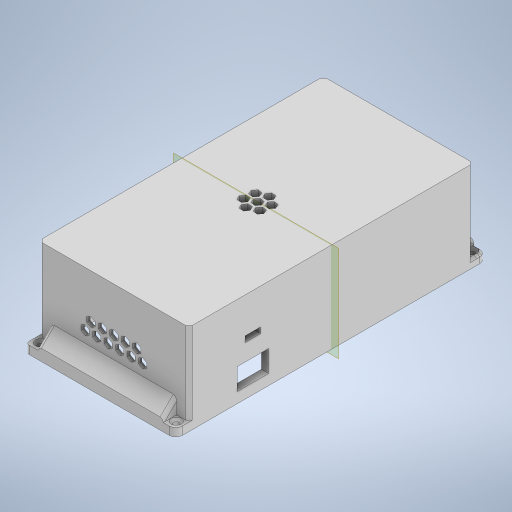
# Autodesk Inventor part: electronics-mount
Saved by Autodesk Inventor 2024.2 (Build 282272000, 272)
## iProperties
Created: 2024-02-05
Part Number: electronics-mount
Material: Generic
Document SubType Name: Modeling
Designer: crow
Density: 1 g/cm^3
Appearance: Default
Author: crow
## iProperties of the stored document electronics-mount_3DPrint.ipt
Created: 2024-02-08
Part Number: electronics-mount_3DPrint
Material: Generic
Document SubType Name: Modeling
Designer: crow
Density: 1 g/cm^3
Appearance: Default
Author: crow
Autodesk Inventor part; units mm, degrees
ref_plane "YZ Plane" through (0, 0, 0) normal (1, 0, 0) x (0, 1, 0)
ref_plane "XZ Plane" through (0, 0, 0) normal (0, 1, 0) x (-1, 0, 0)
ref_plane "XY Plane" through (0, 0, 0) normal (0, 0, 1) x (1, 0, 0)
sketch "Sketch1" plane through (0, 0, 0) normal (0, 1, 0) x (-1, 0, 0)
  line L0 (-41.6915, 94.55) -> (43.6915, 94.55)
  line L1 (45.6915, 92.55) -> (45.6915, -90.55)
  line L2 (41.6915, -94.55) -> (-41.6915, -94.55)
  line L3 (-45.6915, -90.55) -> (-45.6915, 90.55)
  line L4 (41.305, 89.8895) -> (-41.305, 89.8895) construction
  line L5 (0, 89.8895) -> (0, -90.716948) construction
  line L6 (62.379819, 0) -> (-60.787127, 0) construction
  line L7 (41.305, 89.8895) -> (41.305, -89.8895) construction
  line L8 (41.305, 0) -> (-44.332283, 0) construction
  arc A0 (45.6915, 92.55) -> (43.6915, 94.55) centre (43.6915, 92.55) ccw
  arc A1 (41.6915, -94.55) -> (45.6915, -90.55) centre (41.6915, -90.55) ccw
  arc A2 (-45.6915, -90.55) -> (-41.6915, -94.55) centre (-41.6915, -90.55) ccw
  arc A3 (-41.6915, 94.55) -> (-45.6915, 90.55) centre (-41.6915, 90.55) ccw
  line L9 (41.3045, 84.55) -> (-41.3045, 84.55)
  line L10 (-41.3045, 84.55) -> (-41.3045, -84.55)
  line L11 (-41.3045, -84.55) -> (41.3045, -84.55)
  line L12 (41.3045, -84.55) -> (41.3045, 84.55)
  point P0 (0, 0)
  point P1 (45.6915, -94.55)
  point P2 (45.6915, 94.55)
  point P3 (-45.6915, -94.55)
  point P4 (-41.305, -89.8895)
  dimension "d0" = 91.383
  dimension "d1" = 189.1
  dimension "d2" = 82.61
  dimension "d3" = 179.779
  dimension "d4" = 82.61
  dimension "d5" = 2
  dimension "d6" = 4
  dimension "d16" = 10
  dimension "d17" = 4.387
  dimension "d18" = 10
  dimension "d19" = 4.387
  constraints: 26 end point, 8 point on circle, 8 point on line, 8 tangent, 5 horizontal, 4 centre point, 4 parallel, 2 coincident, 2 equal radius, 2 midpoint, 2 perpendicular, 2 vertical
  measures "d0" distance of point (45.691, -94.55) point (-45.691, -94.55)
  measures "d1" distance of point (45.691, 94.55) point (45.691, -94.55)
  measures "d2" distance of L4.start L4.end
  measures "d3" distance of L4.start L7.end
  measures "d4" distance of point (41.305, -89.889) point (-41.305, -89.889)
  measures "d5" radius of A0
  measures "d6" radius of A1
  measures "d16" distance between parallel lines of L0 L9
  measures "d17" distance between parallel lines of L1 L12
  measures "d18" distance between parallel lines of L2 L11
  measures "d19" distance between parallel lines of L3 L10
extrude "Extrusion1" add sketch "Sketch1" against normal blind 5
hole "Hole1" at (-41.305, 0, 89.8895) at (41.305, 0, 89.8895) at (-41.305, 0, -89.8895) at (41.305, 0, -89.8895) direction (0, -1, 0) diameter 3.4 depth 5 countersink diameter 6.3 countersink angle 90 clearance for "Countersunk Flat Head Screw ISO 2009/7046" size "M3" standard "ISO"
sketch "Sketch2" plane through (0, 0, 0) normal (0, 1, 0) x (1, 0, 0)
  line L0 (-41.3045, -84.55) -> (-41.3045, 84.55)
  line L1 (41.3045, -84.55) -> (-41.3045, -84.55)
  line L2 (41.3045, 84.55) -> (41.3045, -84.55)
  line L3 (-41.3045, 84.55) -> (41.3045, 84.55)
  line L4 (-43.6915, -86.55) -> (43.6915, -86.55)
  line L5 (45.6915, -84.55) -> (45.6915, 84.710496)
  line L6 (43.6915, 86.710496) -> (-43.6915, 86.710496)
  line L7 (-45.6915, 84.710496) -> (-45.6915, -84.55)
  line L8 (-43.6915, -86.55) -> (-45.6915, -84.55)
  line L9 (-45.6915, 84.710496) -> (-43.6915, 86.710496)
  line L10 (45.6915, 84.710496) -> (43.6915, 86.710496)
  line L11 (45.6915, -84.55) -> (43.6915, -86.55)
  line L12 (45.6915, -90.55) -> (45.6915, 90.55)
  line L13 (-45.6915, 90.55) -> (-45.6915, -92.55)
  point P0 (0, 0)
  point P1 (-45.6915, -86.55)
  point P2 (-45.6915, 86.710496)
  point P3 (45.6915, 86.710496)
  point P4 (45.6915, -86.55)
  dimension "d20" = 2
  dimension "d24" = 2
  dimension "d25" = 2
  dimension "d26" = 2
  dimension "d27" = 2
  dimension "d28" = 2
  dimension "d29" = 2
  dimension "d30" = 2
  dimension "d31" = 2
  constraints: 16 end point, 8 point on line, 2 collinear
  measures "d20" distance between parallel lines of L1 L4
  measures "d24" distance of L4.start point (-45.692, -86.55)
  measures "d25" distance of L7.end point (-45.692, -86.55)
  measures "d26" distance of L7.start point (-45.692, 86.71)
  measures "d27" distance of L6.end point (-45.692, 86.71)
  measures "d28" distance of L5.end point (45.691, 86.71)
  measures "d29" distance of L6.start point (45.691, 86.71)
  measures "d30" distance of L5.start point (45.691, -86.55)
  measures "d31" distance of L4.end point (45.691, -86.55)
extrude "Extrusion2" add sketch "Sketch2" along normal blind 40
sketch "Sketch3" plane through (0, 40, 0) normal (0, 1, 0) x (1, 0, 0)
  line L0 (-45.6915, -84.55) -> (-43.6915, -86.55)
  line L1 (-43.6915, -86.55) -> (43.6915, -86.55)
  line L2 (43.6915, -86.55) -> (45.6915, -84.55)
  line L3 (45.6915, -84.55) -> (45.6915, 84.710496)
  line L4 (45.6915, 84.710496) -> (43.6915, 86.710496)
  line L5 (43.6915, 86.710496) -> (-43.6915, 86.710496)
  line L6 (-43.6915, 86.710496) -> (-45.6915, 84.710496)
  line L7 (-45.6915, 84.710496) -> (-45.6915, -84.55)
  line L8 (-41.3045, -84.55) -> (-41.3045, 84.55)
  line L9 (-41.3045, 84.55) -> (41.3045, 84.55)
  line L10 (41.3045, 84.55) -> (41.3045, -84.55)
  line L11 (41.3045, -84.55) -> (-41.3045, -84.55)
  point P0 (0, 0)
extrude "Extrusion3" add sketch "Sketch3" along normal blind 10 contours L7 L6 L5 L4 L3 L2 L1 L0 | L8 L9 L10 L11
sketch "Sketch4" plane through (0, 40, 0) normal (0, -1, 0) x (1, 0, 0)
  line L0 (-41.3045, -84.55) -> (-41.3045, 84.55)
  line L1 (-41.3045, 84.55) -> (41.3045, 84.55)
  line L2 (41.3045, -84.55) -> (-41.3045, -84.55)
  line L3 (40.8045, 67.80558) -> (-34.1955, 67.80558)
  line L4 (-34.1955, 67.80558) -> (-34.1955, 29.80558)
  line L5 (-34.1955, 29.80558) -> (40.8045, 29.80558)
  line L6 (40.8045, 29.80558) -> (40.8045, 67.80558)
  line L7 (41.3045, 84.55) -> (41.3045, -84.55)
  circle A0 centre (-29.1955, 62.80558) radius 2
  line L8 (-34.1955, 48.80558) -> (40.8045, 48.80558)
  line L9 (3.3045, 67.80558) -> (3.3045, 29.80558)
  circle A1 centre (-29.1955, 34.80558) radius 2
  line L10 (3.3045, 29.80558) -> (3.3045, 67.80558)
  circle A2 centre (35.8045, 62.80558) radius 2
  circle A3 centre (35.8045, 34.80558) radius 2
  line L11 (29, -27.05) -> (-29, -27.05)
  line L12 (-29, -27.05) -> (-29, -82.55)
  line L13 (-29, -82.55) -> (29, -82.55)
  line L14 (29, -82.55) -> (29, -27.05)
  line L15 (0, -27.05) -> (0, -82.55) construction
  line L16 (-29, -54.8) -> (29, -54.8) construction
  line L17 (0, 99.928537) -> (0, -124.554691) construction
  circle A4 centre (24.5, -37.55) radius 2
  circle A5 centre (24.5, -72.05) radius 2
  circle A6 centre (-15.5, -48.55) radius 2
  circle A7 centre (-15.5, -61.05) radius 2
  line L18 (35, 18.5) -> (-35, 18.5)
  line L19 (-35, 18.5) -> (-35, -18.5)
  line L20 (-35, -18.5) -> (35, -18.5)
  line L21 (35, -18.5) -> (35, 18.5)
  line L22 (0, 18.5) -> (0, -18.5) construction
  line L23 (35, 0) -> (-35, 0) construction
  line L24 (74.043024, 0) -> (-69.253155, 0) construction
  circle A8 centre (0, -25) radius 2
  line L25 (0, -25) -> (0, 25)
  circle A9 centre (0, 25) radius 2
  line L26 (0, 0) -> (13.891236, 0)
  dimension "d123" = 75
  dimension "d124" = 38
  dimension "d125" = 0.5
  dimension "d126" = 4
  dimension "d129" = 58
  dimension "d130" = 55.5
  dimension "d131" = 2
  dimension "d132" = 4
  dimension "d133" = 5
  dimension "d134" = 5
  dimension "d135" = 10.5
  dimension "d136" = 4.5
  dimension "d138" = 4.5
  dimension "d139" = 34.5
  dimension "d140" = 13.5
  dimension "d141" = 21.5
  dimension "d142" = 13.5
  dimension "d143" = 12.5
  dimension "d144" = 70
  dimension "d145" = 37
  dimension "d153" = 4
  dimension "d154" = 50
  dimension "d155" = 4
  constraints: 46 end point, 13 midpoint, 10 centre point, 6 horizontal, 6 parallel, 5 symmetric about line, 4 collinear, 3 equal radius, 3 perpendicular, 2 point on line, 2 vertical, 1 coincident, 3 other
  measures "d123" distance of L5.end L4.end
  measures "d124" distance of L4.end L3.end
  measures "d125" distance between parallel lines of L7 L6
  measures "d126" diameter of A0
  measures "d129" distance of L13.end L12.end
  measures "d130" distance of L12.end L11.end
  measures "d131" distance between parallel lines of L2 L13
  measures "d132" diameter of A4
  measures "d133" distance from line of L3 A0.centre
  measures "d134" distance from line of L4 A0.centre
  measures "d135" distance from line of L11 A4.centre
  measures "d136" distance from line of L14 A4.centre
  measures "d138" distance from line of L14 A5.centre
  measures "d139" distance of A4.centre A5.centre
  measures "d140" distance from line of L12 A6.centre
  measures "d141" distance from line of L11 A6.centre
  measures "d142" distance from line of L12 A7.centre
  measures "d143" distance of A7.centre A6.centre
  measures "d144" distance of L20.end L19.end
  measures "d145" distance of L19.end L18.end
  measures "d153" diameter of A8
  measures "d154" distance of L25.start L25.end
  measures "d155" diameter of A9
extrude "Extrusion4" cut sketch "Sketch4" against normal blind 8.2 contours A0 | A1 | A2 | A3 | A4 | A5 | A6 | A7 | A8 | A9
sketch "Sketch5" plane through (0, 0, 0) normal (0, 1, 0) x (1, 0, 0)
  line L0 (-41.6915, 94.55) -> (41.6915, 94.55) projected
  line L1 (38.155, 94.55) -> (-38.155, 94.55)
  line L2 (-38.155, 94.55) -> (-38.155, 86.7395)
  line L3 (-38.155, 86.7395) -> (38.155, 86.7395)
  line L4 (38.155, 86.7395) -> (38.155, 94.55)
  circle A0 centre (41.305, 89.8895) radius 3.15 projected
  point P0 (0, 0)
  constraints: 8 end point, 2 parallel, 1 horizontal, 1 perpendicular, 1 point on line, 1 tangent
extrude "Extrusion5" add sketch "Sketch5" along normal blind 10 contours L0 L4 L3 L2
chamfer "Chamfer4" distance 7.81 angle 45 1 edges at (0, 10, -94.55)
chamfer "Chamfer5" distance 1.5 angle 45 6 edges at (-45.6915, 0, -87.6302) (-44.5199, 0, -93.3784) (-39.9232, 0, -94.55) (44.5199, 0, -93.3784) (39.9233, 0, -94.55) (45.6915, 0, -87.6302)
fillet "Fillet1" radius 2 2 edges at (38.155, 6.095, -90.645) (-38.155, 6.095, -90.645)
ref_plane "Work Plane2" through (43.6915, 0, -0.080248) normal (0, 0, -1) x (-1, 0, 0)
mirror "Mirror1" about plane through (43.6915, 0, -0.080248) normal (0, 0, -1) of "Extrusion5", "Fillet1", "Chamfer4"
move faces "Move1" translate (0, 0, 0.160496) faces at (12.051667, 0.73, 94.389504)
sketch "Sketch7" plane through (45.6915, -5, 90.55) normal (1, 0, 0) x (0, 0, -1)
  line L0 (175.1, 45) -> (6, 45)
  line L1 (181.1, 0) -> (0, 0)
  line L2 (6, 5) -> (6, 55)
  line L3 (57.74442, 45) -> (53.74442, 45)
  line L4 (29.74442, 45) -> (25.74442, 45)
  line L5 (29.74442, 53.2) -> (25.74442, 53.2)
  line L6 (57.74442, 53.2) -> (53.74442, 53.2)
  line L7 (55.74442, 53.2) -> (55.74442, 64.703518)
  line L8 (27.74442, 53.2) -> (27.74442, 64.703518)
  line L9 (55.74442, 45) -> (55.74442, 35)
  line L10 (55.74442, 35) -> (27.74442, 35)
  line L11 (27.74442, 35) -> (27.74442, 45)
  line L12 (55.74442, 35) -> (55.74442, 33.4)
  line L13 (55.74442, 33.4) -> (27.74442, 33.4)
  line L14 (27.74442, 33.4) -> (27.74442, 35)
  line L15 (47.54442, 29.9) -> (38.24442, 29.9)
  line L16 (38.24442, 29.9) -> (38.24442, 33.4)
  line L17 (38.24442, 33.4) -> (47.54442, 33.4)
  line L18 (47.54442, 33.4) -> (47.54442, 29.9)
  line L19 (52.49442, 19.6) -> (33.29442, 19.6)
  line L20 (33.29442, 19.6) -> (33.29442, 6.4)
  line L21 (33.29442, 6.4) -> (52.49442, 6.4)
  line L22 (52.49442, 6.4) -> (52.49442, 19.6)
  line L23 (42.89442, 6.4) -> (42.89442, 19.6) construction
  line L24 (52.49442, 13) -> (33.29442, 13) construction
  point P0 (90.55, 5)
  point P1 (38.24442, 31.65)
  point P2 (47.54442, 31.65)
  point P3 (47.54442, 33.4)
  point P4 (40, 13)
  point P5 (42.89442, 13)
  point P6 (42.89442, 29.9)
  dimension "d156" = 10
  dimension "d157" = 28
  dimension "d158" = 1.6
  dimension "d160" = 8.2
  dimension "d161" = 9.3
  dimension "d162" = 3.5
  dimension "d166" = 19.2
  dimension "d167" = 13.2
  dimension "d170" = 16.9
  dimension "d171" = 0
  constraints: 36 end point, 12 midpoint, 4 parallel, 4 perpendicular, 4 vertical, 2 collinear, 2 horizontal
  measures "d156" distance of L9.start L9.end
  measures "d157" distance of L9.end L10.end
  measures "d158" distance of L9.end L12.end
  measures "d160" distance from line of L9 point (47.544, 31.65)
  measures "d161" distance of L15.start L15.end
  measures "d162" distance of L15.end L16.end
  measures "d166" distance of L21.end L20.end
  measures "d167" distance of L20.end L19.end
  measures "d170" distance from line of L15 point (42.894, 13)
  measures "d171" distance from line of point (42.894, 29.9) L23
extrude "Extrusion7" cut sketch "Sketch7" against normal blind 10 contours L18 L15 L16 L13 | L22 L21 L20 L19
sketch "Sketch6" plane through (-45.6915, -5, 92.55) normal (-1, 0, 0) x (0, 0, 1)
  circle A0 centre (-44.89442, 13) radius 6.2
  line L0 (-8, 45) -> (-177.1, 45)
  line L1 (-8, 5) -> (-8, 55)
  line L2 (-54.49442, 6.4) -> (-54.49442, 19.6)
  line L3 (-35.29442, 19.6) -> (-35.29442, 6.4)
  line L4 (-35.29442, 6.4) -> (-54.49442, 6.4)
  line L5 (-54.49442, 19.6) -> (-35.29442, 19.6)
  line L6 (-44.89442, 6.4) -> (-44.89442, 19.6) construction
  line L7 (-54.49442, 13) -> (-35.29442, 13) construction
  point P0 (-92.55, 5)
  dimension "d96" = 12.4
  dimension "d97" = 32
  constraints: 5 midpoint, 4 end point, 1 centre point
  measures "d96" diameter of A0
  measures "d97" distance from line of L0 A0.centre
extrude "Extrusion6" cut sketch "Sketch6" against normal blind 10 contours A0
sketch "Sketch8" plane through (0, 50, 0) normal (0, 1, 0) x (1, 0, 0)
  circle A0 centre (-16.5, -72.55) radius 2
  circle A1 centre (16.5, -72.55) radius 2
  line L0 (-43.6915, -86.55) -> (43.6915, -86.55)
  line L1 (43.6915, -86.55) -> (45.6915, -84.55)
  line L2 (45.6915, -84.55) -> (45.6915, 84.710496)
  line L3 (45.6915, 84.710496) -> (43.6915, 86.710496)
  line L4 (43.6915, 86.710496) -> (-43.6915, 86.710496)
  line L5 (-43.6915, 86.710496) -> (-45.6915, 84.710496)
  line L6 (-45.6915, 84.710496) -> (-45.6915, -84.55)
  line L7 (-45.6915, -84.55) -> (-43.6915, -86.55)
  circle A2 centre (16.5, 22.45) radius 2
  circle A3 centre (-16, 22.45) radius 2
  circle A4 centre (-21.7, 43.35) radius 2
  circle A5 centre (-21.7, 74.75) radius 2
  circle A6 centre (19.7, 67.15) radius 2
  circle A7 centre (19.7, 50.95) radius 2
  line L8 (3.494033, -6.426738) -> (1.264827, -9.442376)
  line L9 (1.264827, -9.442376) -> (-2.461396, -9.019647)
  line L10 (-2.461396, -9.019647) -> (-3.958413, -5.581278)
  line L11 (-3.958413, -5.581278) -> (-1.729206, -2.565639)
  line L12 (-1.729206, -2.565639) -> (1.997017, -2.988369)
  line L13 (1.997017, -2.988369) -> (3.494033, -6.426738)
  line L14 (-1.851552, -8.395342) -> (-3.112827, -5.797266)
  line L15 (-3.112827, -5.797266) -> (-1.493465, -3.405931)
  line L16 (-1.493465, -3.405931) -> (1.387173, -3.612673)
  line L17 (1.387173, -3.612673) -> (2.648448, -6.21075)
  line L18 (2.648448, -6.21075) -> (1.029085, -8.602084)
  line L19 (1.029085, -8.602084) -> (-1.851552, -8.395342)
  line L20 (4.226223, 0.02727) -> (2.729206, 3.465639)
  line L21 (2.729206, 3.465639) -> (-0.997017, 3.888369)
  line L22 (-0.997017, 3.888369) -> (-3.226223, 0.87273)
  line L23 (-3.226223, 0.87273) -> (-1.729206, -2.565639)
  line L24 (1.997017, -2.988369) -> (4.226223, 0.02727)
  line L25 (-0.542522, 3.143318) -> (-2.353743, 0.893808)
  line L26 (-2.353743, 0.893808) -> (-1.311221, -1.79951)
  line L27 (-1.311221, -1.79951) -> (1.542522, -2.243318)
  line L28 (1.542522, -2.243318) -> (3.353743, 0.006192)
  line L29 (3.353743, 0.006192) -> (2.311221, 2.69951)
  line L30 (2.311221, 2.69951) -> (-0.542522, 3.143318)
  line L31 (-1.729206, -2.565639) -> (-3.958413, -5.581278)
  line L32 (-2.574792, -2.349651) -> (-4.194154, -4.740985)
  line L33 (-6.716704, 0.455167) -> (-3.836067, 0.248425)
  line L34 (-4.194154, -4.740985) -> (-7.074792, -4.534243)
  line L35 (-3.958413, -5.581278) -> (-7.684636, -5.158548)
  line L36 (-6.952446, 1.29546) -> (-3.226223, 0.87273)
  line L37 (-7.074792, -4.534243) -> (-8.336067, -1.936167)
  line L38 (-8.336067, -1.936167) -> (-6.716704, 0.455167)
  line L39 (-7.684636, -5.158548) -> (-9.181653, -1.720179)
  line L40 (-9.181653, -1.720179) -> (-6.952446, 1.29546)
  line L41 (-3.836067, 0.248425) -> (-2.574792, -2.349651)
  line L42 (-2.494033, 7.326738) -> (-0.997017, 3.888369)
  line L43 (-3.226223, 0.87273) -> (-0.997017, 3.888369)
  line L44 (-8.449463, 4.733829) -> (-6.952446, 1.29546)
  line L45 (-6.53446, 2.061589) -> (-3.680717, 1.617781)
  line L46 (-7.576983, 4.754907) -> (-6.53446, 2.061589)
  line L47 (-3.680717, 1.617781) -> (-1.869497, 3.867291)
  line L48 (-5.765762, 7.004417) -> (-7.576983, 4.754907)
  line L49 (-6.220257, 7.749467) -> (-8.449463, 4.733829)
  line L50 (-1.869497, 3.867291) -> (-2.912019, 6.560609)
  line L51 (-2.912019, 6.560609) -> (-5.765762, 7.004417)
  line L52 (-2.494033, 7.326738) -> (-6.220257, 7.749467)
  line L53 (-0.997017, 3.888369) -> (2.729206, 3.465639)
  line L54 (4.958413, 6.481278) -> (2.729206, 3.465639)
  line L55 (-0.387173, 4.512673) -> (-1.648448, 7.11075)
  line L56 (-2.494033, 7.326738) -> (-0.264827, 10.342376)
  line L57 (-1.648448, 7.11075) -> (-0.029085, 9.502084)
  line L58 (4.112827, 6.697266) -> (2.493465, 4.305931)
  line L59 (-0.029085, 9.502084) -> (2.851552, 9.295342)
  line L60 (-0.264827, 10.342376) -> (3.461396, 9.919647)
  line L61 (2.851552, 9.295342) -> (4.112827, 6.697266)
  line L62 (3.461396, 9.919647) -> (4.958413, 6.481278)
  line L63 (2.493465, 4.305931) -> (-0.387173, 4.512673)
  line L64 (2.729206, 3.465639) -> (4.226223, 0.02727)
  line L65 (7.952446, -0.39546) -> (4.226223, 0.02727)
  line L66 (7.952446, -0.39546) -> (10.181653, 2.620179)
  line L67 (10.181653, 2.620179) -> (8.684636, 6.058548)
  line L68 (7.497952, 0.349591) -> (9.309172, 2.599101)
  line L69 (9.309172, 2.599101) -> (8.26665, 5.292419)
  line L70 (4.644209, 0.793399) -> (7.497952, 0.349591)
  line L71 (8.26665, 5.292419) -> (5.412907, 5.736227)
  line L72 (8.684636, 6.058548) -> (4.958413, 6.481278)
  line L73 (3.601686, 3.486717) -> (4.644209, 0.793399)
  line L74 (5.412907, 5.736227) -> (3.601686, 3.486717)
  line L75 (4.226223, 0.02727) -> (2.729206, 3.465639)
  line L76 (3.494033, -6.426738) -> (7.220257, -6.849467)
  line L77 (7.220257, -6.849467) -> (9.449463, -3.833829)
  line L78 (9.449463, -3.833829) -> (7.952446, -0.39546)
  line L79 (7.952446, -0.39546) -> (4.226223, 0.02727)
  line L80 (4.226223, 0.02727) -> (1.997017, -2.988369)
  line L81 (8.576983, -3.854907) -> (7.53446, -1.161589)
  line L82 (7.53446, -1.161589) -> (4.680717, -0.717781)
  line L83 (4.680717, -0.717781) -> (2.869497, -2.967291)
  line L84 (2.869497, -2.967291) -> (3.912019, -5.660609)
  line L85 (3.912019, -5.660609) -> (6.765762, -6.104417)
  line L86 (6.765762, -6.104417) -> (8.576983, -3.854907)
  point P0 (0, 0)
  point P1 (-0.23219, -6.004008)
  point P2 (-0.23219, -6.004008)
  point P3 (0.5, 0.45)
  point P4 (0.5, 0.45)
  point P5 (-5.455429, -2.142909)
  point P6 (-5.455429, -2.142909)
  point P7 (-4.72324, 4.311099)
  point P8 (-4.72324, 4.311099)
  point P9 (1.23219, 6.904008)
  point P10 (1.23219, 6.904008)
  point P11 (6.455429, 3.042909)
  point P12 (6.455429, 3.042909)
  point P13 (5.72324, -3.411099)
  point P14 (5.72324, -3.411099)
  point P15 (-8.433144, -3.439364)
  point P16 (-3.209904, -7.300462)
  point P17 (-2.48219, -7.096304)
  point P18 (2.01781, -4.911711)
  dimension "d111" = 22
  dimension "d112" = 16
  dimension "d116" = 4.5
  constraints: 158 end point, 66 symmetric about line, 7 coincident, 4 midpoint, 26 other
  measures "d111" vertical distance of A2.centre point (0.5, 0.45)
  measures "d112" horizontal distance of A2.centre point (0.5, 0.45)
  measures "d116" horizontal distance of point (-2.482, -7.096) point (2.018, -4.912)
extrude "Extrusion8" cut sketch "Sketch8" against normal blind 10 contours L14 L15 L16 L17 L18 L19 | L30 L29 L28 L27 L26 L25 | L32 L34 L37 L38 L33 L41 | L46 L48 L51 L50 L47 L45 | L55 L57 L59 L61 L58 L63 | L70 L73 L74 L71 L69 L68 | L86 L85 L84 L83 L82 L81
sketch "Sketch9" plane through (43.6915, 0, -86.710496) normal (0, 0, -1) x (-1, 0, 0)
  line L0 (87.383, 0) -> (87.383, 50) construction
  line L1 (0, 0) -> (0, 50) construction
  line L2 (56.6915, 15.57735) -> (54.1915, 14.133975)
  line L3 (54.1915, 14.133975) -> (51.6915, 15.57735)
  line L4 (51.6915, 15.57735) -> (51.6915, 18.464102)
  line L5 (51.6915, 18.464102) -> (54.1915, 19.907477)
  line L6 (54.1915, 19.907477) -> (56.6915, 18.464102)
  line L7 (56.6915, 18.464102) -> (56.6915, 15.57735)
  line L8 (57.6915, 15) -> (54.1915, 12.979274)
  line L9 (54.1915, 12.979274) -> (50.6915, 15)
  line L10 (50.6915, 15) -> (50.6915, 19.041452)
  line L11 (50.6915, 19.041452) -> (54.1915, 21.062178)
  line L12 (54.1915, 21.062178) -> (57.6915, 19.041452)
  line L13 (57.6915, 19.041452) -> (57.6915, 15)
  line L14 (44.6915, 15.57735) -> (47.1915, 14.133975)
  line L15 (47.1915, 14.133975) -> (49.6915, 15.57735)
  line L16 (49.6915, 15.57735) -> (49.6915, 18.464102)
  line L17 (49.6915, 18.464102) -> (47.1915, 19.907477)
  line L18 (47.1915, 19.907477) -> (44.6915, 18.464102)
  line L19 (44.6915, 18.464102) -> (44.6915, 15.57735)
  line L20 (43.6915, 15) -> (47.1915, 12.979274)
  line L21 (47.1915, 12.979274) -> (50.6915, 15)
  line L22 (50.6915, 19.041452) -> (47.1915, 21.062178)
  line L23 (47.1915, 21.062178) -> (43.6915, 19.041452)
  line L24 (43.6915, 19.041452) -> (43.6915, 15)
  line L25 (36.6915, 15) -> (36.6915, 19.041452)
  line L26 (40.1915, 19.907477) -> (42.6915, 18.464102)
  line L27 (42.6915, 18.464102) -> (42.6915, 15.57735)
  line L28 (43.6915, 15) -> (40.1915, 12.979274)
  line L29 (40.1915, 21.062178) -> (43.6915, 19.041452)
  line L30 (42.6915, 15.57735) -> (40.1915, 14.133975)
  line L31 (37.6915, 18.464102) -> (40.1915, 19.907477)
  line L32 (40.1915, 14.133975) -> (37.6915, 15.57735)
  line L33 (37.6915, 15.57735) -> (37.6915, 18.464102)
  line L34 (40.1915, 12.979274) -> (36.6915, 15)
  line L35 (36.6915, 19.041452) -> (40.1915, 21.062178)
  line L36 (29.6915, 19.041452) -> (29.6915, 15)
  line L37 (35.6915, 15.57735) -> (35.6915, 18.464102)
  line L38 (36.6915, 19.041452) -> (33.1915, 21.062178)
  line L39 (33.1915, 12.979274) -> (36.6915, 15)
  line L40 (33.1915, 14.133975) -> (35.6915, 15.57735)
  line L41 (35.6915, 18.464102) -> (33.1915, 19.907477)
  line L42 (33.1915, 19.907477) -> (30.6915, 18.464102)
  line L43 (33.1915, 21.062178) -> (29.6915, 19.041452)
  line L44 (30.6915, 15.57735) -> (33.1915, 14.133975)
  line L45 (29.6915, 15) -> (33.1915, 12.979274)
  line L46 (30.6915, 18.464102) -> (30.6915, 15.57735)
  line L47 (50.6915, 25.969655) -> (48.1915, 24.526279)
  line L48 (48.1915, 24.526279) -> (48.1915, 21.639528)
  line L49 (48.1915, 21.639528) -> (50.6915, 20.196152)
  line L50 (50.6915, 20.196152) -> (53.1915, 21.639528)
  line L51 (53.1915, 21.639528) -> (53.1915, 24.526279)
  line L52 (53.1915, 24.526279) -> (50.6915, 25.969655)
  line L53 (50.6915, 27.124356) -> (47.1915, 25.10363)
  line L54 (47.1915, 25.10363) -> (47.1915, 21.062178)
  line L55 (47.1915, 21.062178) -> (50.6915, 19.041452)
  line L56 (54.1915, 21.062178) -> (54.1915, 25.10363)
  line L57 (54.1915, 25.10363) -> (50.6915, 27.124356)
  line L58 (43.6915, 19.041452) -> (40.1915, 21.062178)
  line L59 (43.6915, 19.041452) -> (47.1915, 21.062178)
  line L60 (43.6915, 25.969655) -> (46.1915, 24.526279)
  line L61 (46.1915, 24.526279) -> (46.1915, 21.639528)
  line L62 (46.1915, 21.639528) -> (43.6915, 20.196152)
  line L63 (43.6915, 20.196152) -> (41.1915, 21.639528)
  line L64 (41.1915, 21.639528) -> (41.1915, 24.526279)
  line L65 (41.1915, 24.526279) -> (43.6915, 25.969655)
  line L66 (40.1915, 21.062178) -> (40.1915, 25.10363)
  line L67 (40.1915, 25.10363) -> (43.6915, 27.124356)
  line L68 (43.6915, 27.124356) -> (47.1915, 25.10363)
  line L69 (33.1915, 21.062178) -> (36.6915, 19.041452)
  line L70 (40.1915, 21.062178) -> (36.6915, 19.041452)
  line L71 (33.1915, 25.10363) -> (33.1915, 21.062178)
  line L72 (34.1915, 24.526279) -> (34.1915, 21.639528)
  line L73 (36.6915, 25.969655) -> (34.1915, 24.526279)
  line L74 (36.6915, 27.124356) -> (33.1915, 25.10363)
  line L75 (39.1915, 21.639528) -> (39.1915, 24.526279)
  line L76 (39.1915, 24.526279) -> (36.6915, 25.969655)
  line L77 (40.1915, 25.10363) -> (36.6915, 27.124356)
  line L78 (36.6915, 20.196152) -> (39.1915, 21.639528)
  line L79 (34.1915, 21.639528) -> (36.6915, 20.196152)
  line L80 (87.383, 50) -> (0, 50) construction
  line L81 (43.6915, 50) -> (43.6915, 10) construction
  line L82 (79.8465, 10) -> (7.5365, 10) construction
  line L83 (29.6915, 27.124356) -> (33.1915, 25.10363)
  line L84 (29.6915, 20.196152) -> (27.1915, 21.639528)
  line L85 (26.1915, 21.062178) -> (26.1915, 25.10363)
  line L86 (32.1915, 21.639528) -> (29.6915, 20.196152)
  line L87 (27.1915, 21.639528) -> (27.1915, 24.526279)
  line L88 (32.1915, 24.526279) -> (32.1915, 21.639528)
  line L89 (33.1915, 25.10363) -> (33.1915, 21.062178)
  line L90 (29.6915, 25.969655) -> (32.1915, 24.526279)
  line L91 (26.1915, 25.10363) -> (29.6915, 27.124356)
  line L92 (27.1915, 24.526279) -> (29.6915, 25.969655)
  line L93 (29.6915, 19.041452) -> (26.1915, 21.062178)
  line L94 (29.6915, 15) -> (29.6915, 19.041452)
  line L95 (26.1915, 12.979274) -> (29.6915, 15)
  line L96 (23.6915, 18.464102) -> (23.6915, 15.57735)
  line L97 (28.6915, 18.464102) -> (26.1915, 19.907477)
  line L98 (22.6915, 19.041452) -> (22.6915, 15)
  line L99 (26.1915, 14.133975) -> (28.6915, 15.57735)
  line L100 (28.6915, 15.57735) -> (28.6915, 18.464102)
  line L101 (26.1915, 21.062178) -> (22.6915, 19.041452)
  line L102 (26.1915, 19.907477) -> (23.6915, 18.464102)
  line L103 (23.6915, 15.57735) -> (26.1915, 14.133975)
  line L104 (22.6915, 15) -> (26.1915, 12.979274)
  line L105 (57.6915, 19.041452) -> (54.1915, 21.062178)
  line L106 (57.6915, 25.969655) -> (60.1915, 24.526279)
  line L107 (60.1915, 24.526279) -> (60.1915, 21.639528)
  line L108 (60.1915, 21.639528) -> (57.6915, 20.196152)
  line L109 (57.6915, 20.196152) -> (55.1915, 21.639528)
  line L110 (55.1915, 21.639528) -> (55.1915, 24.526279)
  line L111 (55.1915, 24.526279) -> (57.6915, 25.969655)
  line L112 (54.1915, 25.10363) -> (57.6915, 27.124356)
  line L113 (57.6915, 27.124356) -> (61.1915, 25.10363)
  line L114 (61.1915, 25.10363) -> (61.1915, 21.062178)
  line L115 (61.1915, 21.062178) -> (57.6915, 19.041452)
  line L116 (57.6915, 15) -> (57.6915, 19.041452)
  line L117 (57.6915, 15) -> (61.1915, 12.979274)
  line L118 (63.6915, 15.57735) -> (63.6915, 18.464102)
  line L119 (61.1915, 14.133975) -> (63.6915, 15.57735)
  line L120 (58.6915, 15.57735) -> (61.1915, 14.133975)
  line L121 (61.1915, 12.979274) -> (64.6915, 15)
  line L122 (64.6915, 15) -> (64.6915, 19.041452)
  line L123 (63.6915, 18.464102) -> (61.1915, 19.907477)
  line L124 (64.6915, 19.041452) -> (61.1915, 21.062178)
  line L125 (61.1915, 19.907477) -> (58.6915, 18.464102)
  line L126 (58.6915, 18.464102) -> (58.6915, 15.57735)
  point P0 (43.6915, 0)
  point P1 (54.1915, 17.020726)
  point P2 (56.6915, 17.020726)
  point P3 (54.1915, 17.020726)
  point P4 (57.6915, 17.020726)
  point P5 (47.1915, 17.020726)
  point P6 (44.6915, 17.020726)
  point P7 (47.1915, 17.020726)
  point P8 (43.6915, 17.020726)
  point P9 (40.1915, 17.020726)
  point P10 (40.1915, 17.020726)
  point P11 (42.6915, 17.020726)
  point P12 (33.1915, 17.020726)
  point P13 (33.1915, 17.020726)
  point P14 (30.6915, 17.020726)
  point P15 (50.6915, 23.082904)
  point P16 (51.9415, 25.247967)
  point P17 (50.6915, 23.082904)
  point P18 (52.4415, 26.113993)
  point P19 (43.6915, 23.082904)
  point P20 (42.4415, 25.247967)
  point P21 (43.6915, 23.082904)
  point P22 (41.9415, 26.113993)
  point P23 (36.6915, 23.082904)
  point P24 (36.6915, 23.082904)
  point P25 (37.9415, 25.247967)
  point P26 (38.4415, 26.113993)
  point P27 (28.4415, 20.91784)
  point P28 (29.6915, 23.082904)
  point P29 (29.6915, 23.082904)
  point P30 (27.4415, 19.185789)
  point P31 (57.6915, 23.082904)
  point P32 (56.4415, 25.247967)
  point P33 (57.6915, 23.082904)
  point P34 (55.9415, 26.113993)
  point P35 (61.1915, 17.020726)
  point P36 (61.1915, 17.020726)
  dimension "d117" = 5
  dimension "d118" = 1
  dimension "d120" = 5
  constraints: 246 end point, 123 symmetric about line, 10 coincident, 4 midpoint, 1 collinear, 26 other
  measures "d117" distance between parallel lines of L4 L7
  measures "d118" distance between parallel lines of L13 L7
  measures "d120" distance from line of L82 L20.start
extrude "Extrusion9" cut sketch "Sketch9" against normal blind 10 contours L2 L3 L4 L5 L6 L7 | L19 L18 L17 L16 L15 L14 | L26 L27 L30 L32 L33 L31 | L40 L44 L46 L42 L41 L37 | L52 L51 L50 L49 L48 L47 | L60 L61 L62 L63 L64 L65 | L73 L76 L75 L78 L79 L72 | L84 L87 L92 L90 L88 L86 | L102 L97 L100 L99 L103 L96 | L106 L107 L108 L109 L110 L111 | L119 L120 L126 L125 L123 L118
mirror "Mirror2" about plane through (43.6915, 0, -0.080248) normal (0, 0, -1) of "Extrusion9"
equation "\"d4\" = d2"
equation "\"d17\" = d19"
equation "\"d25\" = d24"
equation "\"d26\" = d24"
equation "\"d27\" = d26"
equation "\"d28\" = d24"
equation "\"d29\" = d28"
equation "\"d30\" = d24"
equation "\"d31\" = d30"
body "Solid1"
